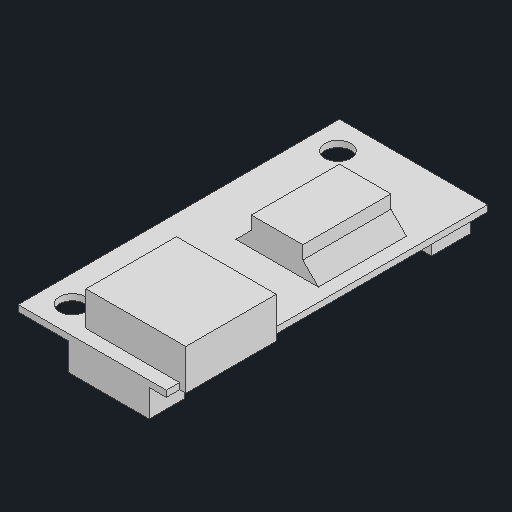
# Autodesk Inventor part: interface_board
Saved by Autodesk Inventor 2023 (Build 270158000, 158)
## iProperties
Created: 2024-04-13
Part Number: interface_board
Material: Generic
Document SubType Name: Modeling
Designer: szymo
Appearance: Default
Surface Area: 19.714 cm^2
Volume: 1.59586 cm^3
Mass: 5 g
Density: 3.13311 g/cm^3
TOTAL MASS: 0.0
Author: szymo
Autodesk Inventor part; units mm, degrees
ref_plane "YZ Plane" through (0, 0, 0) normal (1, 0, 0) x (0, 1, 0)
ref_plane "XZ Plane" through (0, 0, 0) normal (0, 1, 0) x (-1, 0, 0)
ref_plane "XY Plane" through (0, 0, 0) normal (0, 0, 1) x (1, 0, 0)
sketch "Sketch1" plane through (0, 0, 0) normal (0, 1, 0) x (-1, 0, 0)
  line L0 (0, 0) -> (-19, 0)
  line L1 (-19, 0) -> (-19, -41.2)
  line L2 (-19, -41.2) -> (0, -41.2)
  line L3 (0, -41.2) -> (0, 0)
  line L4 (-1.75, 0) -> (-1.75, -41.2)
  line L5 (0, -39.25) -> (-19, -39.25)
  circle A0 centre (-3.425, -3.525) radius 1.675
  circle A1 centre (-3.425, -37.575) radius 1.675
  line L6 (-8.7, -21.2) -> (-15.3, -21.2)
  line L7 (-15.3, -21.2) -> (-15.3, -32.5)
  line L8 (-15.3, -32.5) -> (-8.7, -32.5)
  line L9 (-8.7, -32.5) -> (-8.7, -21.2)
  line L10 (-7, -1.7) -> (-19.8, -1.7)
  line L11 (-19.8, -1.7) -> (-19.8, -13.3)
  line L12 (-19.8, -13.3) -> (-7, -13.3)
  line L13 (-7, -13.3) -> (-7, -1.7)
  line L14 (0, -1.85) -> (-19, -1.85)
  dimension "d0" = 19
  dimension "d1" = 41.2
  dimension "d2" = 1.75
  dimension "d4" = 1.95
  dimension "d5" = 3.35
  dimension "d6" = 3.35
  dimension "d7" = 6.6
  dimension "d8" = 11.3
  dimension "d11" = 8.7
  dimension "d12" = 8.7
  dimension "d13" = 12.8
  dimension "d14" = 11.6
  dimension "d16" = 1.7
  dimension "d27" = 1.85
  dimension "d28" = 7
  constraints: 30 end point, 6 parallel, 6 perpendicular, 6 point on line, 4 tangent, 3 horizontal, 2 centre point
  measures "d0" distance of L2.end L1.end
  measures "d1" distance of L1.end L0.end
  measures "d2" distance between parallel lines of L4 L3
  measures "d4" distance between parallel lines of L5 L2
  measures "d5" diameter of A0
  measures "d6" diameter of A1
  measures "d7" distance of L8.end L7.end
  measures "d8" distance of L7.end L6.end
  measures "d11" distance between parallel lines of L3 L9
  measures "d12" distance between parallel lines of L2 L8
  measures "d13" distance of L11.end L12.end
  measures "d14" distance of L12.end L10.start
  measures "d16" distance between parallel lines of L0 L10
  measures "d27" distance between parallel lines of L0 L14
  measures "d28" distance between parallel lines of L13 L3
extrude "Extrusion1" add sketch "Sketch1" along normal blind 0.8 contours L3 L14 L4 L0 | L4 L14 L13 L10 L1 L0 | L3 L5 L4 L14 | L4 A0 L14 | L3 L2 L4 L5 | L10 L13 L14 L1 | L4 A1 L5 L1 L12 L13 L14 A0 | L5 A1 L4 | L4 L2 L1 L5 | L14 L13 L12 L1 | L9 L8 L7 L6
extrude "Extrusion2" add sketch "Sketch1" along normal blind 5.2 contours L10 L13 L14 L1 | L1 L12 L11 L10 | L14 L13 L12 L1
extrude "Extrusion3" add sketch "Sketch1" along normal blind 4.5 contours L9 L8 L7 L6
chamfer "Chamfer1" distance 2 angle 45 2 edges at (15.3, 0.8, -26.85) (8.7, 0.8, -26.85)
sketch "Sketch2" plane through (0, 0, 0) normal (0, -1, 0) x (1, 0, 0)
  line L0 (19, 0) -> (19, -1.7) projected
  line L1 (0, 0) -> (19, 0) projected
  line L2 (0, -41.2) -> (0, 0) projected
  line L3 (19, -41.2) -> (0, -41.2) projected
  line L4 (19, -13.3) -> (19, -41.2) projected
  line L5 (19.8, -13.3) -> (19, -13.3) projected
  line L6 (19.8, -1.7) -> (19.8, -13.3) projected
  line L7 (19, -1.7) -> (19.8, -1.7) projected
  circle A0 centre (3.425, -3.525) radius 1.675 projected
  circle A1 centre (3.425, -37.575) radius 1.675 projected
  line L8 (0, -41.2) -> (19, -41.2)
  line L9 (19, -41.2) -> (19, 0)
  line L10 (19, 0) -> (0, 0)
  line L11 (0, 0) -> (0, -41.2)
  line L12 (6.4, 0) -> (16.8, 0)
  line L13 (16.8, 0) -> (16.8, -4.5)
  line L14 (16.8, -4.5) -> (6.4, -4.5)
  line L15 (6.4, -4.5) -> (6.4, 0)
  line L16 (9.8, -41.2) -> (16.8, -41.2)
  line L17 (16.8, -41.2) -> (16.8, -36.2)
  line L18 (16.8, -36.2) -> (9.8, -36.2)
  line L19 (9.8, -36.2) -> (9.8, -41.2)
  dimension "d29" = 10.4
  dimension "d30" = 4.5
  dimension "d31" = 0
  dimension "d32" = 6.4
  dimension "d33" = 7
  dimension "d34" = 5
  dimension "d35" = 2.2
  dimension "d36" = 0
  constraints: 24 end point, 6 parallel, 3 horizontal, 3 perpendicular
  measures "d29" distance of L13.end L14.end
  measures "d30" distance of L12.end L13.end
  measures "d31" distance between parallel lines of L10 L12
  measures "d32" distance between parallel lines of L15 L2
  measures "d33" distance of L18.end L17.end
  measures "d34" distance of L17.end L16.end
  measures "d35" distance between parallel lines of L17 L9
  measures "d36" distance between parallel lines of L3 L16
extrude "Extrusion4" add sketch "Sketch2" along normal blind 3.5 contours L13 L14 L15 L1 | L3 L19 L18 L17
body "Solid1"
